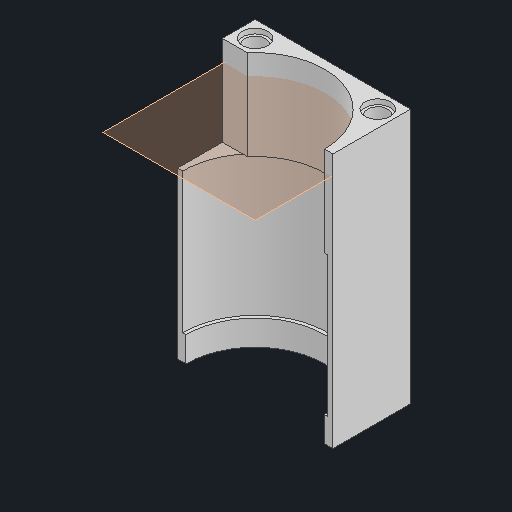
# Autodesk Inventor part: motur_holder
Saved by Autodesk Inventor 2023 (Build 270158000, 158)
## iProperties
Created: 2024-04-29
Part Number: motur_holder
Material: Generic
Document SubType Name: Modeling
Designer: szymo
Density: 1 g/cm^3
Appearance: Default
Mass: 7.85818 g
Surface Area: 56.7462 cm^2
Volume: 7.85818 cm^3
Author: szymo
Autodesk Inventor part; units mm, degrees
ref_plane "YZ Plane" through (0, 0, 0) normal (1, 0, 0) x (0, 1, 0)
ref_plane "XZ Plane" through (0, 0, 0) normal (0, 1, 0) x (-1, 0, 0)
ref_plane "XY Plane" through (0, 0, 0) normal (0, 0, 1) x (1, 0, 0)
ref_plane "Work Plane1" through (25.625, 84.2, 15.375) normal (0, 1, 0) x (0, 0, -1)
sketch "Sketch1" plane through (25.625, 84.2, 15.375) normal (0, 1, 0) x (0, 0, -1)
  line L0 (11.5, -1.5) -> (11, -1.5) projected
  line L1 (11, -1.5) -> (11, 1.5) projected
  line L2 (11, 1.5) -> (11.5, 1.5) projected
  line L3 (11.5, 1.5) -> (11.5, -1.5) projected
  line L4 (-12, -1.5) -> (-12, 1.5) projected
  line L5 (-12, 1.5) -> (-11.5, 1.5) projected
  line L6 (-11.5, 1.5) -> (-11.5, -1.5) projected
  line L7 (-11.5, -1.5) -> (-12, -1.5) projected
  circle A0 centre (0, 0) radius 5 projected
  circle A1 centre (0, 0) radius 13.7 projected
  line L8 (18.875, -15.375) -> (18.875, 116.625) projected
  line L9 (18.875, 116.625) -> (15.375, 116.625) projected
  line L10 (15.375, -15.375) -> (15.375, 116.625) projected
  line L11 (18.875, -15.375) -> (15.375, -15.375) projected
  line L12 (15.375, -15.375) -> (0, -15.375)
  line L13 (0, -15.375) -> (0, 15.375)
  line L14 (0, 15.375) -> (15.375, 15.375)
  line L15 (15.375, 15.375) -> (15.375, -15.375)
  circle A2 centre (12.125, 12.125) radius 3.25
  circle A3 centre (12.125, -12.125) radius 3.25
  line L16 (8.875, 15.375) -> (8.875, 10.4367)
  point P0 (15.375, 25.625)
  point P1 (0, -13.7)
  dimension "d2" = 15.375
  dimension "d3" = 15.375
  dimension "d4" = 6.5
  dimension "d5" = 6.5
  constraints: 10 end point, 5 tangent, 2 centre point, 2 parallel, 2 perpendicular, 1 horizontal, 1 midpoint, 1 point on line, 2 other
  measures "d2" distance of L12.end A0.centre
  measures "d3" distance of L13.end A0.centre
  measures "d4" diameter of A2
  measures "d5" diameter of A3
ref_plane "Work Plane2" through (11.25, 70.4, 1) normal (0, 1, 0) x (0, 0, 1)
extrude "Extrusion1" add sketch "Sketch1" along normal blind 4 and the other way blind 13.8 contours A1 L16 A2 L10 A3 L12 L13 | L16 L14 A2 | A2 | A3 L10 L12 | A3 | L14 L10 A2
sketch "Sketch2" plane through (25.625, 70.4, 15.375) normal (0, -1, 0) x (1, 0, 0)
  arc A0 (-3.651, 5.9062) -> (-4.7619, 7.7035) centre (-4.2064, 6.8048) ccw projected
  arc A1 (-3.651, 5.9062) -> (-6.4477, 2.5768) centre (0, 0) ccw projected
  arc A2 (-8.4097, 3.3608) -> (-6.4477, 2.5768) centre (-7.4287, 2.9688) ccw projected
  arc A3 (-4.7619, 7.7035) -> (-8.4097, 3.3608) centre (0, 0) ccw projected
  arc A4 (6.4477, 2.5768) -> (8.4097, 3.3608) centre (7.4287, 2.9688) ccw projected
  arc A5 (6.4477, 2.5768) -> (3.651, 5.9062) centre (0, 0) ccw projected
  arc A6 (4.7619, 7.7035) -> (3.651, 5.9062) centre (4.2064, 6.8048) ccw projected
  arc A7 (8.4097, 3.3608) -> (4.7619, 7.7035) centre (0, 0) ccw projected
  arc A8 (-6.4563, -2.5553) -> (-8.4209, -3.3328) centre (-7.4386, -2.9441) ccw projected
  arc A9 (-6.4563, -2.5553) -> (-3.651, -5.9062) centre (0, 0) ccw projected
  arc A10 (-4.7619, -7.7035) -> (-3.651, -5.9062) centre (-4.2064, -6.8048) ccw projected
  arc A11 (-8.4209, -3.3328) -> (-4.7619, -7.7035) centre (0, 0) ccw projected
  arc A12 (3.651, -5.9062) -> (4.7619, -7.7035) centre (4.2064, -6.8048) ccw projected
  arc A13 (3.651, -5.9062) -> (6.4563, -2.5553) centre (0, 0) ccw projected
  arc A14 (8.4209, -3.3328) -> (6.4563, -2.5553) centre (7.4386, -2.9441) ccw projected
  arc A15 (4.7619, -7.7035) -> (8.4209, -3.3328) centre (0, 0) ccw projected
  circle A16 centre (10.65, 0.0124) radius 1.15 projected
  circle A17 centre (0, 8) radius 1.0564 projected
  circle A18 centre (0, -8) radius 1.0564 projected
  circle A19 centre (0, 0) radius 5 projected
  circle A20 centre (0, 0) radius 13.7 projected
  line L0 (15.375, -18.875) -> (-116.625, -18.875) projected
  line L1 (-116.625, -18.875) -> (-116.625, -15.375) projected
  line L2 (15.375, -15.375) -> (-116.625, -15.375) projected
  line L3 (15.375, -18.875) -> (15.375, -15.375) projected
  line L4 (15.375, -15.375) -> (-15.375, -15.375)
  line L5 (-15.375, -15.375) -> (-15.375, 0)
  line L6 (-15.375, 0) -> (15.375, 0)
  line L7 (15.375, 0) -> (15.375, -15.375)
  circle A21 centre (0, 0) radius 14.375
  point P0 (-25.625, -15.375)
  point P1 (13.7, 0)
  point P2 (-13.7, 0)
  point P3 (-15.375, -15.375)
  point P4 (14.375, 0)
  point P5 (-14.375, 0)
  dimension "d10" = 15.375
  dimension "d11" = 15.375
  constraints: 8 end point, 2 parallel, 1 centre point, 1 horizontal, 1 midpoint, 1 perpendicular, 2 other
  measures "d10" distance of A1.centre L6.end
  measures "d11" distance of L5.end A1.centre
ref_plane "Work Plane3" through (11.25, 42.7, 1) normal (0, -1, 0) x (1, 0, 0)
extrude "Extrusion2" add sketch "Sketch2" along normal up to surface (27.7 mm away) contours L6 L7 L2 L5 A21
sketch "Sketch3" plane through (25.625, 42.7, 15.375) normal (0, -1, 0) x (1, 0, 0)
  arc A0 (-3.651, 5.9062) -> (-4.7619, 7.7035) centre (-4.2064, 6.8048) ccw projected
  arc A1 (-3.651, 5.9062) -> (-6.4477, 2.5768) centre (0, 0) ccw projected
  arc A2 (-8.4097, 3.3608) -> (-6.4477, 2.5768) centre (-7.4287, 2.9688) ccw projected
  arc A3 (-4.7619, 7.7035) -> (-8.4097, 3.3608) centre (0, 0) ccw projected
  arc A4 (6.4477, 2.5768) -> (8.4097, 3.3608) centre (7.4287, 2.9688) ccw projected
  arc A5 (6.4477, 2.5768) -> (3.651, 5.9062) centre (0, 0) ccw projected
  arc A6 (4.7619, 7.7035) -> (3.651, 5.9062) centre (4.2064, 6.8048) ccw projected
  arc A7 (8.4097, 3.3608) -> (4.7619, 7.7035) centre (0, 0) ccw projected
  arc A8 (-6.4563, -2.5553) -> (-8.4209, -3.3328) centre (-7.4386, -2.9441) ccw projected
  arc A9 (-6.4563, -2.5553) -> (-3.651, -5.9062) centre (0, 0) ccw projected
  arc A10 (-4.7619, -7.7035) -> (-3.651, -5.9062) centre (-4.2064, -6.8048) ccw projected
  arc A11 (-8.4209, -3.3328) -> (-4.7619, -7.7035) centre (0, 0) ccw projected
  arc A12 (3.651, -5.9062) -> (4.7619, -7.7035) centre (4.2064, -6.8048) ccw projected
  arc A13 (3.651, -5.9062) -> (6.4563, -2.5553) centre (0, 0) ccw projected
  arc A14 (8.4209, -3.3328) -> (6.4563, -2.5553) centre (7.4386, -2.9441) ccw projected
  arc A15 (4.7619, -7.7035) -> (8.4209, -3.3328) centre (0, 0) ccw projected
  circle A16 centre (10.65, 0.0124) radius 1.15 projected
  circle A17 centre (0, 8) radius 1.0564 projected
  circle A18 centre (0, -8) radius 1.0564 projected
  circle A19 centre (0, 0) radius 5 projected
  circle A20 centre (0, 0) radius 13.7 projected
  line L0 (15.375, -18.875) -> (-116.625, -18.875) projected
  line L1 (-116.625, -18.875) -> (-116.625, -15.375) projected
  line L2 (15.375, -15.375) -> (-116.625, -15.375) projected
  line L3 (15.375, -18.875) -> (15.375, -15.375) projected
  line L4 (15.375, 0) -> (15.375, -15.375) projected
  line L5 (15.375, -15.375) -> (-15.375, -15.375)
  line L6 (-15.375, -15.375) -> (-15.375, 0)
  line L7 (-15.375, 0) -> (15.375, 0)
  line L8 (15.375, 0) -> (15.375, -15.375)
  point P0 (-25.625, -15.375)
  point P1 (15.375, 0)
  point P2 (13.7, 0)
  point P3 (-13.7, 0)
  point P4 (-15.375, -15.375)
  dimension "d14" = 15.375
  dimension "d15" = 15.375
  constraints: 8 end point, 2 parallel, 1 horizontal, 1 midpoint, 1 perpendicular, 1 other
  measures "d14" distance of L7.end A1.centre
  measures "d15" distance of L6.end A1.centre
ref_plane "Work Plane4" through (11.925, 37.7, 1.675) normal (0, -1, 0) x (1, 0, 0)
extrude "Extrusion3" add sketch "Sketch3" along normal up to surface (5 mm away) contours L7 L4 L2 L6 A20
sketch "Sketch4" plane through (25.625, 37.7, 15.375) normal (0, -1, 0) x (1, 0, 0)
  circle A0 centre (-12.125, -12.125) radius 1.8 projected
  circle A1 centre (12.125, -12.125) radius 1.8 projected
  point P0 (-25.625, -15.375)
  constraints: 2 coincident
hole "Hole1" at (13.5, 37.7, 3.25) at (37.75, 37.7, 3.25) direction (0, 1, 0) diameter 4 depth 4.6 counterbore diameter 4.6 counterbore depth 0.6
sketch "Sketch5" plane through (25.625, 88.2, 15.375) normal (0, 1, 0) x (1, 0, 0)
  arc A0 (13.7, 0) -> (-10.4367, 8.875) centre (0, 0) ccw projected
  line L0 (13.7, 0) -> (15.375, 0) projected
  line L1 (15.375, 0) -> (15.375, 15.375) projected
  line L2 (15.375, 15.375) -> (-15.375, 15.375) projected
  line L3 (-15.375, 15.375) -> (-15.375, 8.875) projected
  line L4 (-15.375, 8.875) -> (-10.4367, 8.875) projected
  circle A1 centre (12.125, 12.125) radius 3.25
  circle A2 centre (-12.125, 12.125) radius 3.25
  point P0 (-25.625, 15.375)
  dimension "d25" = 6.5
  dimension "d26" = 6.5
  constraints: 4 tangent, 2 centre point, 2 coincident
  measures "d25" diameter of A1
  measures "d26" diameter of A2
hole "Hole2" at (37.75, 88.2, 3.25) at (13.5, 88.2, 3.25) direction (0, -1, 0) diameter 4 depth 9 counterbore diameter 5 counterbore depth 1
equation "\"d3\" = d2"
equation "\"d11\" = d10"
equation "\"d15\" = d14"
body "Solid1"
